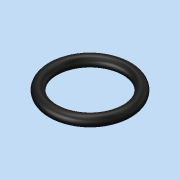
# Autodesk Inventor part: outerORing
Saved by Autodesk Inventor 2017 (Build 210142000, 142)
## iProperties
Created: 2016-10-25
Part Number: outerORing
Material: Generic
Document SubType Name: Modeling
Designer: techn
Density: 1 g/cm^3
Appearance: Glossy - Black
Author: techn
Autodesk Inventor part; units mm, degrees
ref_plane "YZ Plane" through (0, 0, 0) normal (1, 0, 0) x (0, 1, 0)
ref_plane "XZ Plane" through (0, 0, 0) normal (0, 1, 0) x (-1, 0, 0)
ref_plane "XY Plane" through (0, 0, 0) normal (0, 0, 1) x (1, 0, 0)
sketch "Sketch2" plane through (0, 0, 0) normal (0, 0, 1) x (1, 0, 0)
  circle A0 centre (3.5, 0) radius 0.5
  line L0 (3, 0) -> (0, 0)
  line L1 (0, 0) -> (0, 2.7044)
  dimension "d0" = 1
  dimension "d1" = 3
  constraints: 4 end point, 1 horizontal, 1 horizontal alignment, 1 vertical, 2 other
  measures "d1" distance of L0.start L0.end
revolve "Revolution1" add sketch "Sketch2" angle 360 about axis through (0, 0, 0) along (0, 1, 0)
body "Solid1"
